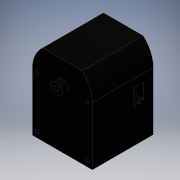
# Autodesk Inventor part: Servo
Saved by Autodesk Inventor 2016 (Build 200138000, 138)
## iProperties
Created: 2015-09-12
Part Number: Servo
Material: プラスチック、不透明 黒
Document SubType Name: Modeling
Designer: daisuke
Density: 0.952 g/cm^3
Appearance: 滑らか - 黒
Mass: 40.3625 g
Surface Area: 92.1098 cm^2
Volume: 42.3976 cm^3
Author: daisuke
Autodesk Inventor part; units mm, degrees
ref_plane "YZ Plane" through (0, 0, 0) normal (1, 0, 0) x (0, 1, 0)
ref_plane "XZ Plane" through (0, 0, 0) normal (0, 1, 0) x (-1, 0, 0)
ref_plane "XY Plane" through (0, 0, 0) normal (0, 0, 1) x (1, 0, 0)
sketch "スケッチ1" plane through (0, 0, 0) normal (0, 1, 0) x (-1, 0, 0)
  line L0 (0, 0) -> (32, 0)
  line L1 (32, 0) -> (32, -43)
  line L2 (32, -43) -> (0, -43)
  line L3 (0, -43) -> (0, 0)
  dimension "d0" = 32
  dimension "d1" = 43
  constraints: 8 end point, 2 parallel, 1 horizontal, 1 perpendicular
  measures "d0" distance of L1.end L2.end
  measures "d1" distance of L0.end L1.end
extrude "押し出し1" add sketch "スケッチ1" along normal blind 32.5
sketch "スケッチ2" plane through (0, 0, 0) normal (0, -1, 0) x (1, 0, 0)
  line L0 (-32, -43) -> (-32, 0) construction
  line L1 (-32, -21.5) -> (0, -21.5) construction
  line L2 (0, 0) -> (0, -43) construction
  line L3 (-16, -21.5) -> (-16, -12) construction
  line L4 (-32, 0) -> (-32, -43) projected
  arc A0 (-26.583, 0) -> (-32, -12) centre (-16, -12) ccw
  arc A1 (0, -12) -> (-5.417, 0) centre (-16, -12) ccw
  line L5 (-32, -12) -> (-32, 0)
  line L6 (0, 0) -> (-32, 0) projected
  line L7 (-5.417, 0) -> (0, 0)
  line L8 (0, 0) -> (0, -12)
  line L9 (-32, 0) -> (-26.583, 0)
  dimension "d4" = 9.5
  constraints: 12 end point, 5 point on circle, 3 collinear, 3 midpoint, 2 centre point, 2 coincident, 2 point on line, 2 tangent, 1 perpendicular, 1 vertical
  measures "d4" distance of L3.start L3.end
extrude "押し出し2" cut sketch "スケッチ2" against normal blind 32.5
sketch "スケッチ3" plane through (0, 0, 0) normal (0, -1, 0) x (1, 0, 0)
  line L0 (-32, -21.5) -> (0, -21.5) construction
  line L1 (0, -21.5) -> (0, -43) construction
  line L2 (-5.417, 0) -> (-26.583, 0) construction
  line L3 (-16, 0) -> (-16, -43) construction
  line L4 (-32, -43) -> (0, -43) construction
  line L5 (-16, -21.5) -> (-16, -13) construction
  line L6 (-16, -21.5) -> (-29.5, -21.5) construction
  circle A0 centre (-29.5, -13) radius 1
  line L7 (-16, -21.5) -> (-2.5, -21.5) construction
  circle A1 centre (-2.5, -13) radius 1
  line L8 (-16, -21.5) -> (-16, -40) construction
  circle A2 centre (-29.5, -40) radius 1
  circle A3 centre (-2.5, -40) radius 1
  point P0 (0, 0)
  dimension "d8" = 8.5
  dimension "d9" = 13.5
  dimension "d10" = 2
  dimension "d11" = 13.5
  dimension "d12" = 2
  dimension "d13" = 18.5
  dimension "d14" = 2
  dimension "d15" = 2
  constraints: 14 end point, 4 centre point, 4 point on line, 3 midpoint
  measures "d8" distance of L5.start L5.end
  measures "d9" distance of L5.start L6.end
  measures "d10" diameter of A0
  measures "d11" distance of L5.start L7.end
  measures "d12" diameter of A1
  measures "d13" distance of L5.start L8.end
  measures "d14" diameter of A2
  measures "d15" diameter of A3
extrude "押し出し3" cut sketch "スケッチ3" against normal blind 32.5
sketch "スケッチ4" plane through (0, 32.5, 0) normal (0, 1, 0) x (1, 0, 0)
  line L0 (-5.417, 0) -> (-26.583, 0) construction
  line L1 (-32, 21.5) -> (0, 21.5) construction
  line L2 (0, 21.5) -> (0, 43) construction
  line L3 (-16, 0) -> (-16, 43) construction
  line L4 (-32, 43) -> (0, 43) construction
  line L5 (-16, 21.5) -> (-16, 13) construction
  line L6 (-16, 21.5) -> (-29.5, 21.5) construction
  circle A0 centre (-29.5, 13) radius 1
  line L7 (-16, 21.5) -> (-2.5, 21.5) construction
  circle A1 centre (-2.5, 13) radius 1
  line L8 (-16, 21.5) -> (-16, 40) construction
  circle A2 centre (-29.5, 40) radius 1
  circle A3 centre (-2.5, 40) radius 1
  line L9 (-29.5, 21.5) -> (-29.5, 22) construction
  line L10 (-2.5, 21.5) -> (-2.5, 35) construction
  line L11 (-16, 21.5) -> (-16, 4.5) construction
  line L12 (-16, 4.5) -> (-5, 4.5) construction
  line L13 (-16, 4.5) -> (-27, 4.5) construction
  circle A4 centre (-2.5, 35) radius 1
  circle A5 centre (-29.5, 22) radius 1
  circle A6 centre (-27, 4.5) radius 1
  circle A7 centre (-5, 4.5) radius 1
  line L14 (0, 43) -> (-32, 43) projected
  line L15 (0, 43) -> (-32, 43)
  line L16 (-32, 43) -> (-32, 12) projected
  line L17 (-32, 43) -> (-32, 12)
  line L18 (0, 12) -> (0, 43) projected
  line L19 (0, 43) -> (0, 12)
  line L20 (-26.583, 0) -> (-5.417, 0) projected
  line L21 (-5.417, 0) -> (-26.583, 0)
  arc A8 (-32, 12) -> (-26.583, 0) centre (-16, 12) ccw
  arc A9 (-5.417, 0) -> (0, 12) centre (-16, 12) ccw projected
  arc A10 (-5.417, 0) -> (0, 12) centre (-16, 12) ccw
  point P0 (0, 0)
  point P1 (0, 0)
  dimension "d26" = 0.5
  dimension "d27" = 13.5
  dimension "d28" = 17
  dimension "d29" = 11
  dimension "d30" = 11
  dimension "d31" = 2
  dimension "d32" = 2
  dimension "d33" = 2
  dimension "d34" = 2
  constraints: 36 end point, 10 centre point, 5 point on line, 4 coincident, 4 point on circle, 3 collinear, 3 vertical, 2 perpendicular, 1 midpoint, 1 tangent
  measures "d26" distance of L6.end L9.end
  measures "d27" distance of L7.end L10.end
  measures "d28" distance of L6.start L11.end
  measures "d29" distance of L11.end L12.end
  measures "d30" distance of L11.end L13.end
  measures "d31" diameter of A4
  measures "d32" diameter of A5
  measures "d33" diameter of A6
  measures "d34" diameter of A7
extrude "押し出し4" cut sketch "スケッチ4" against normal blind 30 contours A4 | A5 | A6 | A7
sketch "スケッチ5" plane through (0, 0, 0) normal (0, -1, 0) x (1, 0, 0)
  line L0 (-32, -21.5) -> (0, -21.5) construction
  line L1 (0, -21.5) -> (0, -43) construction
  line L2 (-5.417, 0) -> (-26.583, 0) construction
  line L3 (-16, 0) -> (-16, -43) construction
  line L4 (-32, -43) -> (0, -43) construction
  line L5 (-16, -21.5) -> (-16, -12) construction
  line L6 (-16, -21.5) -> (-29.5, -21.5) construction
  circle A0 centre (-29.5, -13) radius 1
  line L7 (-16, -21.5) -> (-2.5, -21.5) construction
  circle A1 centre (-2.5, -13) radius 1
  line L8 (-16, -21.5) -> (-16, -40) construction
  circle A2 centre (-29.5, -40) radius 1
  circle A3 centre (-2.5, -40) radius 1
  circle A4 centre (-16, -12) radius 3
  point P0 (0, 0)
  point P1 (0, 0)
  dimension "d37" = 9.5
  dimension "d38" = 13.5
  dimension "d39" = 2
  dimension "d40" = 13.5
  dimension "d41" = 2
  dimension "d42" = 18.5
  dimension "d43" = 2
  dimension "d44" = 2
  dimension "d45" = 6
  constraints: 18 end point, 5 centre point, 4 point on line, 3 midpoint, 1 coincident
  measures "d37" distance of L5.start L5.end
  measures "d38" distance of L5.start L6.end
  measures "d39" diameter of A0
  measures "d40" distance of L5.start L7.end
  measures "d41" diameter of A1
  measures "d42" distance of L5.start L8.end
  measures "d43" diameter of A2
  measures "d44" diameter of A3
  measures "d45" diameter of A4
extrude "押し出し5" add sketch "スケッチ5" along normal blind 3 contours A4
sketch "スケッチ6" plane through (-16, -3, -12) normal (0, -1, 0) x (1, 0, 0)
  circle A0 centre (0, 0) radius 1.3
  point P0 (16, 12)
  dimension "d48" = 2.6
  constraints: 1 centre point
  measures "d48" diameter of A0
extrude "押し出し6" cut sketch "スケッチ6" against normal blind 7
sketch "スケッチ7" plane through (0, 32.5, 0) normal (0, 1, 0) x (1, 0, 0)
  line L0 (-5.417, 0) -> (-26.583, 0) construction
  line L1 (-16, 21.5) -> (-29.5, 21.5) construction
  line L2 (-16, 21.5) -> (-16, 13) construction
  line L3 (-16, 21.5) -> (-2.5, 21.5) construction
  line L4 (-32, 21.5) -> (0, 21.5) construction
  line L5 (-32, 43) -> (0, 43) construction
  line L6 (-16, 21.5) -> (-16, 40) construction
  line L7 (0, 21.5) -> (0, 43) construction
  line L8 (-16, 0) -> (-16, 43) construction
  line L9 (-29.5, 21.5) -> (-29.5, 22) construction
  line L10 (-16, 21.5) -> (-16, 12) construction
  line L11 (-16, 12) -> (-5, 12) construction
  line L12 (-16, 12) -> (-27, 12) construction
  circle A0 centre (-16, 12) radius 1.3 projected
  circle A1 centre (-16, 12) radius 4.25
  point P0 (0, 0)
  point P1 (0, 0)
  point P2 (0, 0)
  dimension "d53" = 9.5
  dimension "d60" = 8.5
  constraints: 26 end point, 5 point on line, 2 perpendicular, 1 centre point, 1 coincident, 1 midpoint, 1 vertical
  measures "d53" distance of L1.start L10.end
  measures "d60" diameter of A1
extrude "押し出し7" cut sketch "スケッチ7" against normal blind 0.5 contours A0 | A1
sketch "スケッチ8" plane through (-16, 32, -12) normal (0, 1, 0) x (1, 0, 0)
  circle A0 centre (0, 0) radius 2.7
  point P0 (16, -12)
  dimension "d63" = 5.4
  constraints: 1 centre point
  measures "d63" diameter of A0
extrude "押し出し8" add sketch "スケッチ8" along normal blind 0.5
sketch "スケッチ9" plane through (-16, 32.5, -12) normal (0, 1, 0) x (1, 0, 0)
  circle A0 centre (0, 0) radius 1.3
  point P0 (16, -12)
  dimension "d66" = 2.6
  constraints: 1 centre point
  measures "d66" diameter of A0
extrude "押し出し9" cut sketch "スケッチ9" against normal blind 10
sketch "スケッチ10" plane through (0, 0, -43) normal (1, 0, 0) x (0, 0, -1)
  line L0 (0, 0) -> (0, 32.5) construction
  line L1 (0, 16.25) -> (-21.5, 16.25) construction
  line L2 (-22, 32.5) -> (-20, 32.5) construction
  line L3 (0, 0) -> (-31, 0) construction
  line L4 (-21, 32.5) -> (-21, 27.5) construction
  line L5 (-21, 27.5) -> (-26.7, 27.5)
  line L6 (-26.7, 27.5) -> (-26.7, 24.6)
  line L7 (-26.7, 24.6) -> (-18, 24.6)
  line L8 (-18, 24.6) -> (-18, 25.6)
  line L9 (-18, 25.6) -> (-19, 25.6)
  line L10 (-19, 25.6) -> (-19, 27.5)
  line L11 (-19, 27.5) -> (-21, 27.5)
  line L12 (-26.7, 24.6) -> (-26.7, 22.1)
  line L13 (-26.7, 22.1) -> (-18, 22.1)
  line L14 (-18, 22.1) -> (-18, 23.1)
  line L15 (-18, 23.1) -> (-19, 23.1)
  line L16 (-19, 23.1) -> (-19, 24.6)
  point P0 (-43, 0)
  dimension "d69" = 21.5
  dimension "d71" = 5
  dimension "d72" = 2.9
  dimension "d73" = 5.7
  dimension "d74" = 8.7
  dimension "d75" = 1
  dimension "d76" = 1
  dimension "d79" = 2.5
  dimension "d80" = 1
  dimension "d81" = 1
  constraints: 28 end point, 8 perpendicular, 3 horizontal, 2 midpoint, 2 vertical, 1 point on line
  measures "d69" distance of L1.start L1.end
  measures "d71" distance of L4.start L4.end
  measures "d72" distance of L5.end L6.end
  measures "d73" distance of L4.end L5.end
  measures "d74" distance of L6.end L7.end
  measures "d75" distance of L7.end L8.end
  measures "d76" distance of L8.end L9.end
  measures "d79" distance of L6.end L12.end
  measures "d80" distance of L13.end L14.end
  measures "d81" distance of L14.end L15.end
extrude "押し出し10" cut sketch "スケッチ10" against normal blind 5
